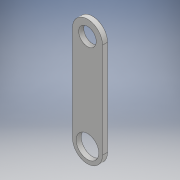
# Autodesk Inventor part: FEMUR
Saved by Autodesk Inventor 2017 (Build 210142000, 142)
## iProperties
Created: 2017-09-24
Part Number: FEMUR
Material: Generic
Document SubType Name: Modeling
Designer: Alexander Miller
Density: 1 g/cm^3
Appearance: Default
Author: Alexander Miller
Autodesk Inventor part; units mm, degrees
ref_plane "YZ Plane" through (0, 0, 0) normal (1, 0, 0) x (0, 1, 0)
ref_plane "XZ Plane" through (0, 0, 0) normal (0, 1, 0) x (-1, 0, 0)
ref_plane "XY Plane" through (0, 0, 0) normal (0, 0, 1) x (1, 0, 0)
sketch "Sketch1" plane through (0, 0, 0) normal (0, 1, 0) x (-1, 0, 0)
  line L0 (6, 25) -> (-6, 25)
  line L1 (-6, 25) -> (-6, -25)
  line L2 (-6, -25) -> (6, -25)
  line L3 (6, -25) -> (6, 25)
  point P0 (0, 0)
  point P1 (0, -25)
  point P2 (6, 0)
  dimension "d0" = 12
  dimension "d1" = 50
  constraints: 8 end point, 2 midpoint, 2 parallel, 1 horizontal, 1 horizontal alignment, 1 perpendicular, 1 vertical alignment
  measures "d0" distance of L1.end L2.end
  measures "d1" distance of L2.end L0.start
extrude "Extrusion1" add sketch "Sketch1" along normal blind 2
full round fillet "Fillet1" first side at (-6, 0.6667, -8.3333) centre faces at (-2, 0.6667, 25) second side at (6, 0.6667, 8.3333)
full round fillet "Fillet2" first side at (6, 1.3333, 4.3334) centre faces at (2, 0.6667, -25) second side at (-6, 0.6667, -10.3333)
sketch "Sketch2" plane through (0, 2, 0) normal (0, 1, 0) x (1, 0, 0)
  circle A0 centre (0, 19) radius 4.5
  circle A1 centre (0, -19) radius 3.5
  arc A2 (6, 19) -> (-6, 19) centre (0, 19) ccw projected
  arc A3 (-6, -19) -> (6, -19) centre (0, -19) ccw projected
  point P0 (0, 0)
  dimension "d4" = 9
  dimension "d5" = 7
  constraints: 2 centre point, 2 concentric
  measures "d4" diameter of A0
  measures "d5" diameter of A1
extrude "Extrusion2" cut sketch "Sketch2" against normal through all
equation "\"d0\" = servo_B"
equation "\"servo_B\" = 12"
body "Solid1"
